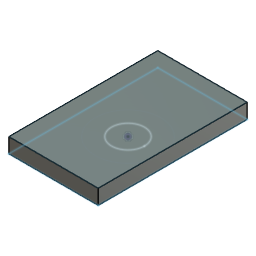
base bar (Autodesk Fusion 360 design; units mm, degrees)
part number: 2026-06-03-15-20-48-513
Autodesk Fusion 360 part; units mm, degrees
sketch "Sketch1" plane through (0, 0, 0) normal (0, 1, 0) x (1, 0, 0)
  line L0 (-45, 75) -> (-45, -75)
  line L1 (-45, -75) -> (45, -75)
  line L2 (45, -75) -> (45, 75)
  line L3 (45, 75) -> (-45, 75)
  circle A0 centre (0, 0) radius 16.5
  dimension "d9" = 33
  constraint perpendicular L0 L1
  constraint perpendicular L1 L2
  constraint coincident A0.centre origin
  measures "d9" diameter of A0
extrude "Extrude1" add sketch "Sketch1" along normal blind 15 contours L0 L1 L2 L3 | A0
move_face "MoveFace1" by (-220, 0, 0) 1 faces at (-15, 15, -25)
sketch "Sketch2" plane through (0, 15, 0) normal (0, 1, 0) x (-1, 0, 0)
  line L0 (-45, -75) -> (45, -75)
  line L1 (45, -75) -> (45, 75)
  line L2 (45, 75) -> (-45, 75)
  line L3 (-45, 75) -> (-45, -75)
sketch "Sketch3" plane through (0, 15, 0) normal (0, 1, 0) x (-1, 0, 0)
  line L0 (-45, -75) -> (45, -75)
  line L1 (45, -75) -> (45, 75)
  line L2 (45, 75) -> (-45, 75)
  line L3 (-45, 75) -> (-45, -75)
sketch "Sketch6" plane through (0, 30, 0) normal (0, 1, 0) x (-1, 0, 0)
sketch "Sketch10" plane through (0, 15, 0) normal (0, 1, 0) x (-1, 0, 0)
combine "Combine1" [no effect]
sketch "Sketch7" plane through (0, 15, 0) normal (0, 1, 0) x (-1, 0, 0)
sketch "Sketch8" plane through (0, 15, 0) normal (0, 1, 0) x (-1, 0, 0)
sketch "Sketch9" plane through (0, 15, 0) normal (0, 1, 0) x (-1, 0, 0)
extrude "Extrude3" [suppressed]
sketch "Sketch4" plane through (0, 0, 0) normal (0, 1, 0) x (1, 0, 0)
sketch "Sketch5" plane through (0, 0, 0) normal (0, 1, 0) x (1, 0, 0)
named bodies: "Body 1"
